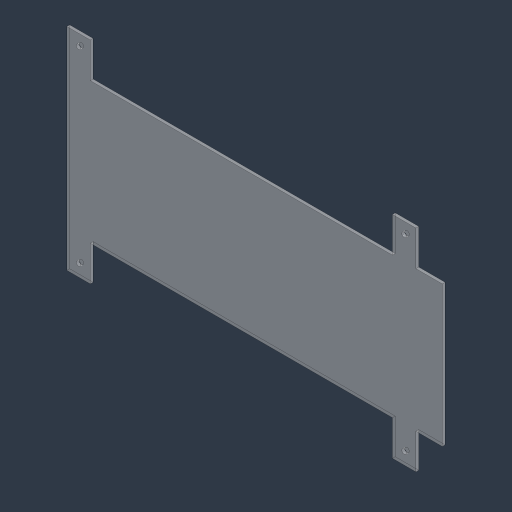
# Autodesk Inventor part: feeder_slide_plate
Saved by Autodesk Inventor 2024.3 (Build 283343000, 343)
## iProperties
Created: 2025-03-09
Part Number: feeder_slide_plate
Material: Polycarbonate, Clear
Document SubType Name: Sheet Metal
Designer: marcu
Density: 1.2 g/cm^3
Sheet Metal Rule: Default
Appearance: Polycarbonate - Clear
Author: marcu
Autodesk Inventor part; units mm, degrees
ref_plane "YZ Plane" through (0, 0, 0) normal (1, 0, 0) x (0, 1, 0)
ref_plane "XZ Plane" through (0, 0, 0) normal (0, 1, 0) x (-1, 0, 0)
ref_plane "XY Plane" through (0, 0, 0) normal (0, 0, 1) x (1, 0, 0)
sketch "Sketch1" plane through (0, 0, 0) normal (0, 0, 1) x (1, 0, 0)
  line L0 (203.2, -76.2) -> (-203.2, -76.2)
  line L1 (-203.2, -76.2) -> (-203.2, 76.2)
  line L2 (-203.2, 76.2) -> (203.2, 76.2)
  line L3 (203.2, 76.2) -> (203.2, -76.2)
  line L4 (203.2, -76.2) -> (-203.2, 76.2) construction
  line L5 (-203.2, -76.2) -> (203.2, 76.2) construction
  line L6 (149.225, -76.2) -> (174.625, -76.2)
  line L7 (174.625, -76.2) -> (174.625, -114.3)
  line L8 (174.625, -114.3) -> (149.225, -114.3)
  line L9 (149.225, -114.3) -> (149.225, -76.2)
  line L10 (0, 0) -> (203.2, 0) construction
  line L11 (174.625, 76.2) -> (174.625, 114.3)
  line L12 (174.625, 114.3) -> (149.225, 114.3)
  line L13 (149.225, 114.3) -> (149.225, 76.2)
  line L14 (-203.2, -76.2) -> (-177.8, -76.2)
  line L15 (-177.8, -76.2) -> (-177.8, -114.3)
  line L16 (-177.8, -114.3) -> (-203.2, -114.3)
  line L17 (-203.2, -114.3) -> (-203.2, -76.2)
  line L18 (149.225, -114.3) -> (149.225, -76.2)
  line L19 (-177.8, 76.2) -> (-177.8, 114.3)
  line L20 (-177.8, 114.3) -> (-203.2, 114.3)
  line L21 (-203.2, 114.3) -> (-203.2, 76.2)
  dimension "d0" = 406.4
  dimension "d1" = 152.4
  dimension "d2" = 25.4
  dimension "d3" = 38.1
  dimension "d4" = 28.575
  dimension "d6" = 25.4
  dimension "d7" = 38.1
  measures "d0" distance of L1.end L2.end
  measures "d1" distance of L0.end L1.end
  measures "d2" distance of L7.end L8.end
  measures "d3" distance of L6.end L7.end
  measures "d4" distance between parallel lines of L3 L7
  measures "d6" distance of L15.end L16.end
  measures "d7" distance of L14.end L15.end
extrude "Plate1" add sketch "Sketch1" along normal blind 3.048
sketch "Sketch2" plane through (0, 0, 3.048) normal (0, 0, 1) x (1, 0, 0)
  line L0 (-203.2, -114.3) -> (-203.2, 114.3) construction
  line L1 (-177.8, -114.3) -> (-203.2, -114.3) construction
  line L2 (-177.8, -76.2) -> (-177.8, -114.3) construction
  line L3 (149.225, -76.2) -> (-177.8, -76.2) construction
  line L4 (149.225, -114.3) -> (149.225, -76.2) construction
  line L5 (174.625, -114.3) -> (149.225, -114.3) construction
  line L6 (174.625, -76.2) -> (174.625, -114.3) construction
  line L7 (203.2, -76.2) -> (174.625, -76.2) construction
  line L8 (203.2, 76.2) -> (203.2, -76.2) construction
  line L9 (174.625, 76.2) -> (203.2, 76.2) construction
  line L10 (174.625, 114.3) -> (174.625, 76.2) construction
  line L11 (149.225, 114.3) -> (174.625, 114.3) construction
  line L12 (149.225, 76.2) -> (149.225, 114.3) construction
  line L13 (-177.8, 76.2) -> (149.225, 76.2) construction
  line L14 (-177.8, 114.3) -> (-177.8, 76.2) construction
  line L15 (-203.2, 114.3) -> (-177.8, 114.3) construction
  point P0 (0, 0)
  point P1 (-190.5, 101.6)
  point P2 (161.925, 101.6)
  point P3 (-190.5, -101.6)
  point P4 (161.925, -101.6)
  dimension "d8" = 12.7
  dimension "d9" = 12.7
  dimension "d12" = 352.425
  dimension "d15" = 203.2
  constraints: 1 horizontal, 1 vertical, 3 other
  measures "d8" distance from line of L15 point (-190.5, 101.6)
  measures "d9" distance from line of L14 point (-190.5, 101.6)
  measures "d12" distance of point (-190.5, 101.6) point (161.925, 101.6)
  measures "d15" distance of point (-190.5, 101.6) point (-190.5, -101.6)
hole "Hole1" at (-190.5, 101.6, 3.048) at (161.925, 101.6, 3.048) at (-190.5, -101.6, 3.048) at (161.925, -101.6, 3.048) direction (0, 0, -1) diameter 5.1054 end through all clearance for "Flat Head Machine Screw (82)" size "#10" standard "Ansi Unified Screw Threads"
equation "\"d23\" = Thickness"
equation "\"d5\" = Thickness"
equation "\"BendRadius\" = Thickness"
equation "\"BendReliefWidth\" = Thickness"
equation "\"BendReliefDepth\" = 0.5 * Thickness"
equation "\"CornerReliefSize\" = 4 * Thickness"
equation "\"MinimumRemnant\" = 2 * Thickness"
equation "\"TransitionRadius\" = BendRadius"
equation "\"JacobiRadiusSize\" = BendRadius"
equation "\"GapSize\" = Thickness"
equation "\"Thickness\" = 3.048"
body "Solid1"
